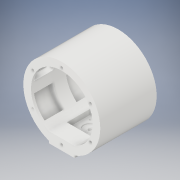
# Autodesk Inventor part: SJ003
Saved by Autodesk Inventor 2017 SP1 (Build 210196100, 196)
## iProperties
Created: 2017-06-01
Part Number: SJ003
Material: ABS Plastic
Document SubType Name: Modeling
Designer: Zach
Density: 1.06 g/cm^3
Appearance: CR White
Author: Zach
Autodesk Inventor part; units mm, degrees
ref_plane "YZ Plane" through (0, 0, 0) normal (1, 0, 0) x (0, 1, 0)
ref_plane "XZ Plane" through (0, 0, 0) normal (0, 1, 0) x (-1, 0, 0)
ref_plane "XY Plane" through (0, 0, 0) normal (0, 0, 1) x (1, 0, 0)
sketch "Sketch1" plane through (0, 0, 0) normal (0, 0, 1) x (1, 0, 0)
  circle A0 centre (0, 0) radius 75
  circle A1 centre (0, 0) radius 60
  dimension "d0" = 150
  dimension "d1" = 15
  constraints: 2 centre point, 1 coincident
  measures "d0" diameter of A0
  measures "d1" radial gap between concentric circles of A0 A1
extrude "Extrusion1" add sketch "Sketch1" along normal mid plane 110
sketch "Sketch3" plane through (0, 0, 55) normal (0, 0, 1) x (1, 0, 0)
  line L0 (25, -54.5436) -> (25, -75)
  line L1 (25, -75) -> (-25, -75)
  line L2 (-25, -75) -> (-25, -54.5436)
  line L3 (-25, -54.5436) -> (25, -54.5436)
  circle A0 centre (0, 0) radius 75 projected
  circle A1 centre (0, 0) radius 60 projected
  circle A2 centre (0, 0) radius 75 projected
  circle A3 centre (0, 0) radius 60 projected
  point P0 (0, -75)
  dimension "d17" = 25
  dimension "d18" = 50
  constraints: 8 end point, 2 perpendicular, 1 horizontal, 1 midpoint, 1 vertical, 1 vertical alignment, 3 other
  measures "d17" horizontal distance of L2.end point (0, 0)
  measures "d18" distance of L2.end L0.start
extrude "Extrusion3" add sketch "Sketch3" against normal blind 110 contours A1 L3 | L0 A0 L2 A1 | L0 L1 A0 | L1 L2 A0 picked at (-5.1003, -55.7011) picked at (0, -64.8523)
sketch "Sketch2" plane through (0, 0, 55) normal (0, 0, 1) x (1, 0, 0)
  circle A0 centre (0, 65) radius 2.5
  circle A1 centre (-56.2917, 32.5) radius 2.5
  circle A2 centre (-56.2917, -32.5) radius 2.5
  circle A3 centre (0, -65) radius 2.5
  circle A4 centre (56.2917, -32.5) radius 2.5
  circle A5 centre (56.2917, 32.5) radius 2.5
  point P0 (0, 0)
  dimension "d4" = 5
  dimension "d5" = 65
  dimension "d8" = 360
  constraints: 6 centre point, 13 other
  measures "d4" diameter of A0
  measures "d5" distance of point (0, 0) A0.centre
extrude "Extrusion2" cut sketch "Sketch2" against normal through all
sketch "Sketch5" plane through (-25, -54.5436, 55) normal (0, 1, 0) x (1, 0, 0)
  line L0 (2.5, 77.5) -> (47.5, 77.5)
  line L1 (47.5, 77.5) -> (47.5, 32.5)
  line L2 (47.5, 32.5) -> (2.5, 32.5)
  line L3 (2.5, 32.5) -> (2.5, 77.5)
  line L4 (2.5, 77.5) -> (47.5, 32.5) construction
  line L5 (47.5, 77.5) -> (2.5, 32.5) construction
  line L6 (0, 0) -> (50, 0) projected
  line L7 (0, 0) -> (0, 110) projected
  line L8 (50, 110) -> (0, 110) projected
  line L9 (50, 0) -> (50, 110) projected
  point P0 (25, 55)
  dimension "d20" = 45
  dimension "d21" = 45
  dimension "d57" = 55
  dimension "d58" = 2.5
  constraints: 12 end point, 2 midpoint, 2 parallel, 1 horizontal, 1 perpendicular
  measures "d20" distance of L1.end L2.end
  measures "d21" distance of L0.end L1.end
  measures "d57" distance from line of L8 point (25, 55)
  measures "d58" distance between parallel lines of L3 L7
extrude "Extrusion4" cut sketch "Sketch5" against normal blind 10 contours L0 L1 L2 L3
sketch "Sketch6" plane through (-25, -64.5436, 55) normal (0, 1, 0) x (1, 0, 0)
  line L0 (39.1421, 40.8579) -> (10.8579, 40.8579) construction
  line L1 (10.8579, 40.8579) -> (10.8579, 69.1421) construction
  line L2 (10.8579, 69.1421) -> (39.1421, 69.1421) construction
  line L3 (39.1421, 69.1421) -> (39.1421, 40.8579) construction
  line L4 (39.1421, 40.8579) -> (10.8579, 69.1421) construction
  line L5 (10.8579, 40.8579) -> (39.1421, 69.1421) construction
  circle A0 centre (10.8579, 69.1421) radius 1.65
  circle A1 centre (39.1421, 69.1421) radius 1.65
  circle A2 centre (39.1421, 40.8579) radius 1.65
  circle A3 centre (10.8579, 40.8579) radius 1.65
  circle A4 centre (25, 55) radius 3
  dimension "d24" = 28.2843
  dimension "d25" = 28.2843
  dimension "d26" = 3.3
  dimension "d27" = 3.3
  dimension "d28" = 3.3
  dimension "d29" = 3.3
  dimension "d32" = 6
  constraints: 12 end point, 5 centre point, 5 coincident, 2 midpoint, 2 parallel, 1 horizontal, 1 perpendicular
  measures "d24" distance of L0.end L1.end
  measures "d25" distance of L1.end L2.end
  measures "d26" diameter of A0
  measures "d27" diameter of A1
  measures "d28" diameter of A2
  measures "d29" diameter of A3
  measures "d32" diameter of A4
extrude "Extrusion5" cut sketch "Sketch6" against normal through all
sketch "Sketch7" plane through (-25, -75, 55) normal (0, -1, 0) x (1, 0, 0)
  line L0 (0, 0) -> (50, 0)
  line L1 (0, 0) -> (0, -120)
  line L2 (50, -120) -> (0, -120)
  line L3 (50, 0) -> (50, -120)
  circle A0 centre (10.8579, -40.8579) radius 1.65
  line L4 (8.6928, -39.6079) -> (10.8579, -38.3579)
  line L5 (10.8579, -38.3579) -> (13.0229, -39.6079)
  line L6 (13.0229, -39.6079) -> (13.0229, -42.1079)
  line L7 (13.0229, -42.1079) -> (10.8579, -43.3579)
  line L8 (10.8579, -43.3579) -> (8.6928, -42.1079)
  line L9 (8.6928, -42.1079) -> (8.6928, -39.6079)
  line L10 (8.6928, -67.8921) -> (10.8579, -66.6421)
  line L11 (10.8579, -66.6421) -> (13.0229, -67.8921)
  line L12 (13.0229, -67.8921) -> (13.0229, -70.3921)
  line L13 (13.0229, -70.3921) -> (10.8579, -71.6421)
  line L14 (10.8579, -71.6421) -> (8.6928, -70.3921)
  line L15 (8.6928, -70.3921) -> (8.6928, -67.8921)
  line L16 (36.9771, -67.8921) -> (39.1421, -66.6421)
  line L17 (39.1421, -66.6421) -> (41.3072, -67.8921)
  line L18 (41.3072, -67.8921) -> (41.3072, -70.3921)
  line L19 (41.3072, -70.3921) -> (39.1421, -71.6421)
  line L20 (39.1421, -71.6421) -> (36.9771, -70.3921)
  line L21 (36.9771, -70.3921) -> (36.9771, -67.8921)
  circle A1 centre (39.1421, -40.8579) radius 1.65
  line L22 (41.3072, -39.6079) -> (41.3072, -42.1079)
  line L23 (41.3072, -42.1079) -> (39.1421, -43.3579)
  line L24 (39.1421, -43.3579) -> (36.9771, -42.1079)
  line L25 (36.9771, -42.1079) -> (36.9771, -39.6079)
  line L26 (36.9771, -39.6079) -> (39.1421, -38.3579)
  line L27 (39.1421, -38.3579) -> (41.3072, -39.6079)
  circle A2 centre (10.8579, -40.8579) radius 1.65 projected
  circle A3 centre (39.1421, -69.1421) radius 1.65 projected
  circle A4 centre (10.8579, -69.1421) radius 1.65 projected
  circle A5 centre (39.1421, -40.8579) radius 1.65 projected
  circle A6 centre (25, -55) radius 3 projected
  line L28 (0, 0) -> (50, 0) projected
  line L29 (0, 0) -> (0, -110) projected
  line L30 (50, -110) -> (0, -110) projected
  line L31 (50, 0) -> (50, -110) projected
  point P0 (25, -60)
  constraints: 56 end point, 6 coincident, 4 vertical alignment, 2 centre point, 1 point on line, 1 vertical, 52 other
extrude "Extrusion6" cut sketch "Sketch7" against normal blind 5 contours A0 | L4 L5 L6 L7 L8 L9 | L10 L11 L12 L13 L14 L15 | L16 L17 L18 L19 L20 L21 | A1 | L22 L23 L24 L25 L26 L27 | A3 | A4
sketch "Sketch8" plane through (-25, -64.5436, 55) normal (0, 1, 0) x (1, 0, 0)
  circle A0 centre (25, 55) radius 12.5
  dimension "d38" = 25
  constraints: 1 centre point, 1 coincident
  measures "d38" diameter of A0
extrude "Extrusion7" cut sketch "Sketch8" against normal blind 2
sketch "Sketch9" plane through (0, 0, 0) normal (0, 0, 1) x (1, 0, 0)
  circle A0 centre (0, 0) radius 70 construction
  line L0 (43.8748, -54.5436) -> (-43.8748, -54.5436)
  arc A1 (43.8748, -54.5436) -> (-43.8748, -54.5436) centre (0, 0) ccw
  point P0 (22.5, -54.5436)
  dimension "d42" = 140
  constraints: 4 point on circle, 2 centre point, 2 concentric, 2 end point, 1 coincident, 1 horizontal, 1 point on line
  measures "d42" diameter of A0
extrude "Extrusion8" cut sketch "Sketch9" along normal mid plane 100
sketch "Sketch10" plane through (0, 0, 0) normal (0, 0, 1) x (1, 0, 0)
  arc A0 (25, -70.7107) -> (-25, -70.7107) centre (0, 0) ccw projected
  arc A1 (73.8606, -13.0236) -> (73.8606, 13.0236) centre (0, 0) ccw
  arc A2 (25, -54.5436) -> (-25, -54.5436) centre (0, 0) ccw projected
  arc A3 (59.0885, -10.4189) -> (59.0885, 10.4189) centre (0, 0) ccw
  line L0 (73.8606, 13.0236) -> (59.0885, 10.4189)
  line L1 (73.8606, -13.0236) -> (59.0885, -10.4189)
  arc A4 (25, -70.7107) -> (-25, -70.7107) centre (0, 0) ccw construction
  line L2 (73.8606, 13.0236) -> (0, 0) construction
  line L3 (0, 0) -> (73.8606, -13.0236) construction
  line L4 (0, 0) -> (147.5691, 0) construction
  line L5 (25.6515, 70.4769) -> (20.5212, 56.3816)
  arc A5 (38.5673, 45.9627) -> (20.5212, 56.3816) centre (0, 0) ccw
  line L6 (48.2091, 57.4533) -> (38.5673, 45.9627)
  arc A6 (48.2091, 57.4533) -> (25.6515, 70.4769) centre (0, 0) ccw
  line L7 (-48.2091, 57.4533) -> (-38.5673, 45.9627)
  arc A7 (-20.5212, 56.3816) -> (-38.5673, 45.9627) centre (0, 0) ccw
  line L8 (-25.6515, 70.4769) -> (-20.5212, 56.3816)
  arc A8 (-25.6515, 70.4769) -> (-48.2091, 57.4533) centre (0, 0) ccw
  line L9 (-73.8606, -13.0236) -> (-59.0885, -10.4189)
  arc A9 (-59.0885, 10.4189) -> (-59.0885, -10.4189) centre (0, 0) ccw
  line L10 (-73.8606, 13.0236) -> (-59.0885, 10.4189)
  arc A10 (-73.8606, 13.0236) -> (-73.8606, -13.0236) centre (0, 0) ccw
  line L11 (-25.6515, -70.4769) -> (-20.5212, -56.3816)
  arc A11 (-38.5673, -45.9627) -> (-20.5212, -56.3816) centre (0, 0) ccw
  line L12 (-48.2091, -57.4533) -> (-38.5673, -45.9627)
  arc A12 (-48.2091, -57.4533) -> (-25.6515, -70.4769) centre (0, 0) ccw
  line L13 (48.2091, -57.4533) -> (38.5673, -45.9627)
  arc A13 (20.5212, -56.3816) -> (38.5673, -45.9627) centre (0, 0) ccw
  line L14 (25.6515, -70.4769) -> (20.5212, -56.3816)
  arc A14 (25.6515, -70.4769) -> (48.2091, -57.4533) centre (0, 0) ccw
  dimension "d45" = 20
  dimension "d48" = 360
  constraints: 30 end point, 29 point on circle, 12 centre point, 2 concentric, 2 point on line, 1 horizontal, 62 other
  measures "d45" angle of L1 L0
extrude "Extrusion9" add sketch "Sketch10" along normal mid plane 100 contours L14 A13 A2 L13 A0 | L1 A2 L0 A0 | L6 A2 L5 A0 | L8 A2 L7 A0 | L10 A2 L9 A0 | L12 A2 A11 L11 A0
sketch "Sketch11" plane through (0, 0, 0) normal (0, 0, 1) x (1, 0, 0)
  arc A0 (25, -70.7107) -> (-25, -70.7107) centre (0, 0) ccw
  line L0 (-51.4782, -54.5436) -> (51.4782, -54.5436) construction
  line L1 (-25, -54.5436) -> (25, -54.5436)
  arc A1 (51.4782, -54.5436) -> (-51.4782, -54.5436) centre (0, 0) ccw
  arc A2 (25, -54.5436) -> (-25, -54.5436) centre (0, 0) ccw
  arc A3 (25, -54.5436) -> (-25, -54.5436) centre (0, 0) ccw
  line L2 (-51.4782, -54.5436) -> (-25, -54.5436)
  line L3 (25, -54.5436) -> (51.4782, -54.5436)
  line L4 (-22.5, -54.5436) -> (22.5, -54.5436)
  constraints: 10 end point, 10 point on circle, 4 centre point, 2 collinear, 2 point on line, 1 concentric
extrude "Extrusion10" add sketch "Sketch11" along normal mid plane 25 contours L3 A2 L2 A0
sketch "Sketch12" plane through (-25, -54.5436, 55) normal (0, 1, 0) x (1, 0, 0)
  line L0 (47.5, 32.5) -> (27.458, 32.5) projected
  line L1 (2.5, 77.5) -> (2.5, 32.5) projected
  line L2 (47.5, 32.5) -> (2.5, 32.5)
  line L3 (2.5, 32.5) -> (2.5, 77.5)
  line L4 (2.5, 77.5) -> (47.5, 77.5)
  line L5 (47.5, 77.5) -> (47.5, 32.5)
  point P0 (25, 55)
  constraints: 8 end point, 2 parallel, 1 horizontal, 1 perpendicular
extrude "Extrusion11" cut sketch "Sketch12" against normal blind 10
body "Solid1"
